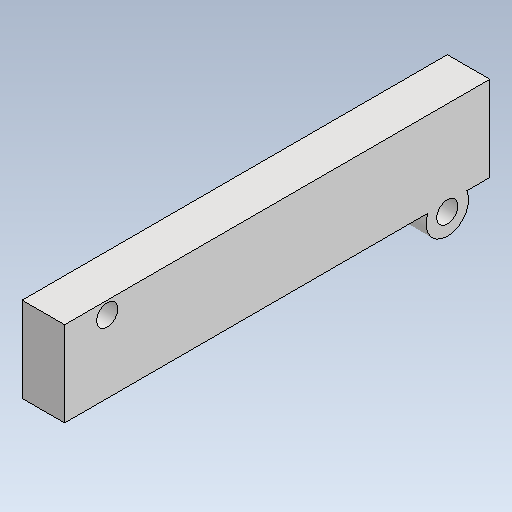
# Autodesk Inventor part: temp-bed
Saved by Autodesk Inventor 2025 (Build 290162000, 162)
## iProperties
Created: 2025-08-20
Part Number: temp-bed
Material: Generic
Document SubType Name: Modeling
Designer: HP
Density: 1 g/cm^3
Appearance: Default
Author: HP
Autodesk Inventor part; units mm, degrees
ref_plane "YZ Plane" through (0, 0, 0) normal (1, 0, 0) x (0, 1, 0)
ref_plane "XZ Plane" through (0, 0, 0) normal (0, 1, 0) x (-1, 0, 0)
ref_plane "XY Plane" through (0, 0, 0) normal (0, 0, 1) x (1, 0, 0)
sketch "Sketch1" plane through (0, 0, 0) normal (1, 0, 0) x (0, 1, 0)
  line L0 (-10, 50) -> (10, 50)
  line L1 (10, 50) -> (10, -50)
  line L2 (10, -50) -> (-10, -50)
  line L3 (-10, -50) -> (-10, 50)
  line L4 (-10, 50) -> (10, -50) construction
  line L5 (10, 50) -> (-10, -50) construction
  circle A0 centre (7, 40) radius 2.5
  circle A1 centre (7, 40) radius 5
  circle A2 centre (-12, -40) radius 2.5
  circle A3 centre (-12, -40) radius 5
  point P0 (0, 0)
  point P1 (0, 0)
  point P2 (-10, 35.4174)
  point P3 (-10, -35.4174)
  point P4 (-10, -44.5826)
  point P5 (-10, 44.5826)
  point P6 (10, 36)
  point P7 (10, 44)
  point P8 (-10, -38.5)
  point P9 (-10, -41.5)
  dimension "d0" = 100
  dimension "d1" = 5
  dimension "d2" = 10
  dimension "d3" = 10
  dimension "d5" = 20
  dimension "d6" = 5
  dimension "d7" = 10
  dimension "d8" = 2
  dimension "d9" = 10
  dimension "d12" = 3
  constraints: 12 end point, 4 centre point, 3 coincident, 2 midpoint, 2 parallel, 1 horizontal, 1 perpendicular
  measures "d0" distance between parallel lines of L2 L0
  measures "d1" diameter of A0
  measures "d2" diameter of A1
  measures "d3" distance from line of L0 A0.centre
  measures "d5" distance between parallel lines of L3 L1
  measures "d6" diameter of A2
  measures "d7" diameter of A3
  measures "d8" distance from line of L3 A2.centre
  measures "d9" distance from line of L2 A2.centre
  measures "d12" distance from line of A0.centre L1
extrude "Extrusion1" add sketch "Sketch1" along normal blind 10 contours L0 L1 A1 L2 L3 A3 | A3 L3 A2 | L3 A2 A3 | L1 A1 picked at (9.8333, 40)
body "Solid1"
